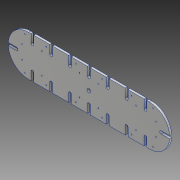
# Autodesk Inventor part: 1313_Former Bottom_V1
Saved by Autodesk Inventor 2020 (Build 240168000, 168)
## iProperties
Created: 2019-09-10
Part Number: 1313_Former Bottom_V1
Material: Aluminum 6061
Document SubType Name: Modeling
Designer: MPI
Density: 2.7 g/cm^3
Appearance: Aluminum - Flat
Mass: 5622.53 g
Surface Area: 6914.04 cm^2
Volume: 5622.53 cm^3
Author: MPI
Autodesk Inventor part; units mm, degrees
ref_plane "Work Plane2" through (0, 0, 0) normal (0, -1, 0) x (1, 0, 0)
sketch "Sketch2" plane through (0, 0, 0) normal (0, -1, 0) x (1, 0, 0)
  line L0 (-432, -146) -> (432, -146)
  line L1 (432, 146) -> (-432, 146)
  line L2 (432, -86) -> (-432, -86) projected
  line L3 (-432, 86) -> (432, 86) projected
  arc A0 (-432, 86) -> (-432, -86) centre (-432, 0) ccw projected
  arc A1 (432, -86) -> (432, 86) centre (432, 0) ccw projected
  arc A2 (432, -146) -> (432, 146) centre (432, 0) ccw
  arc A3 (-432, 146) -> (-432, -146) centre (-432, 0) ccw
  point P0 (0, 0)
  point P1 (480, -91)
  point P2 (480, 91)
  dimension "d11" = 60
  dimension "d12" = 60
  constraints: 4 end point, 4 point on circle, 2 centre point, 2 coincident, 2 tangent, 1 horizontal, 1 parallel, 3 other
extrude "Extrusion2" add sketch "Sketch2" along normal blind 15 contours A3 L1 A2 L0 | L2 A0 L3 A1
ref_plane "Work Plane1" through (0, 7.01, 0) normal (0, 1, 0) x (1, 0, 0)
sketch "Sketch4" plane through (0, 7.01, 0) normal (0, 1, 0) x (1, 0, 0)
  line L0 (-659.0781, -10) -> (-659.0781, 10)
  line L1 (670.9769, 10) -> (670.9769, -10)
  line L2 (-10, 220.6364) -> (10, 220.6364)
  line L3 (-125, -216.3636) -> (-145, -216.3636)
  line L4 (-145, 220.6364) -> (-125, 220.6364)
  line L5 (-260, -216.3636) -> (-280, -216.3636)
  line L6 (-280, 220.6364) -> (-260, 220.6364)
  line L7 (145, -216.3636) -> (125, -216.3636)
  line L8 (125, 220.6364) -> (145, 220.6364)
  line L9 (280, -216.3636) -> (260, -216.3636)
  line L10 (260, 220.6364) -> (280, 220.6364)
  line L11 (395, 220.6364) -> (415, 220.6364)
  line L12 (-432, -86) -> (432, -86) projected
  line L13 (432, 86) -> (-432, 86) projected
  line L14 (395, 86) -> (395, 220.6364)
  line L15 (415, 220.6364) -> (415, 86)
  line L16 (280, -86) -> (280, -216.3636)
  line L17 (260, -216.3636) -> (260, -86)
  line L18 (280, 220.6364) -> (280, 86)
  line L19 (260, 86) -> (260, 220.6364)
  line L20 (145, -86) -> (145, -216.3636)
  line L21 (125, -216.3636) -> (125, -86)
  line L22 (145, 220.6364) -> (145, 86)
  line L23 (125, 86) -> (125, 220.6364)
  line L24 (10, 220.6364) -> (10, 86)
  line L25 (-10, 86) -> (-10, 220.6364)
  line L26 (-125, -86) -> (-125, -216.3636)
  line L27 (-145, -216.3636) -> (-145, -86)
  line L28 (-125, 220.6364) -> (-125, 86)
  line L29 (-145, 86) -> (-145, 220.6364)
  line L30 (-260, -86) -> (-260, -216.3636)
  line L31 (-280, -216.3636) -> (-280, -86)
  line L32 (-260, 220.6364) -> (-260, 86)
  line L33 (-280, 86) -> (-280, 220.6364)
  arc A0 (395, 86) -> (415, 86) centre (405, 86) ccw
  arc A1 (260, 86) -> (280, 86) centre (270, 86) ccw
  arc A2 (125, 86) -> (145, 86) centre (135, 86) ccw
  arc A3 (-10, 86) -> (10, 86) centre (0, 86) ccw
  arc A4 (-145, 86) -> (-125, 86) centre (-135, 86) ccw
  arc A5 (-280, 86) -> (-260, 86) centre (-270, 86) ccw
  arc A6 (-260, -86) -> (-280, -86) centre (-270, -86) ccw
  arc A7 (-125, -86) -> (-145, -86) centre (-135, -86) ccw
  arc A8 (145, -86) -> (125, -86) centre (135, -86) ccw
  arc A9 (280, -86) -> (260, -86) centre (270, -86) ccw
  arc A10 (432, -86) -> (432, 86) centre (432, 0) ccw projected
  arc A11 (518, 10) -> (518, -10) centre (518, 0) ccw
  arc A12 (-518, -10) -> (-518, 10) centre (-518, 0) ccw
  line L34 (-659.0781, 10) -> (-518, 10)
  line L35 (517.4166, 10) -> (670.9769, 10)
  line L36 (670.9769, -10) -> (518, -10)
  line L37 (-518, -10) -> (-659.0781, -10)
  circle A13 centre (-480, 48) radius 3.57
  circle A14 centre (-337.5, 76) radius 3.57
  circle A15 centre (337.5, 76) radius 3.57
  circle A16 centre (480, 48) radius 3.57
  circle A17 centre (480, -48) radius 3.57
  circle A18 centre (337.5, -76) radius 3.57
  circle A19 centre (-337.5, -76) radius 3.57
  circle A20 centre (-480, -48) radius 3.57
  arc A21 (-432, 86) -> (-432, -86) centre (-432, 0) ccw projected
  line L38 (10, -86) -> (10, -216.3636)
  line L39 (-10, -216.3636) -> (-10, -86)
  arc A22 (10, -86) -> (-10, -86) centre (0, -86) ccw
  line L40 (-10, -216.3636) -> (10, -216.3636)
  line L41 (-415, 220.6364) -> (-395, 220.6364)
  line L42 (-395, 220.6364) -> (-395, 86)
  line L43 (-415, 86) -> (-415, 220.6364)
  arc A23 (-415, 86) -> (-395, 86) centre (-405, 86) ccw
  line L44 (415, -216.3636) -> (395, -216.3636)
  line L45 (415, -86) -> (415, -216.3636)
  line L46 (395, -216.3636) -> (395, -86)
  arc A24 (415, -86) -> (395, -86) centre (405, -86) ccw
  line L47 (-395, -216.3636) -> (-415, -216.3636)
  line L48 (-395, -86) -> (-395, -216.3636)
  line L49 (-415, -216.3636) -> (-415, -86)
  arc A25 (-395, -86) -> (-415, -86) centre (-405, -86) ccw
  line L50 (-432, 0) -> (-518, 0)
  circle A26 centre (-67.5, 76) radius 3.57
  circle A27 centre (67.5, 76) radius 3.57
  circle A28 centre (67.5, -76) radius 3.57
  circle A29 centre (-67.5, -76) radius 3.57
  point P0 (480, -91)
  point P1 (480, 91)
  point P2 (-395, 86)
  point P3 (-395, 86)
  dimension "d18" = 20
  dimension "d54" = 76
  dimension "d55" = 48
  dimension "d59" = 48
  dimension "d60" = 76
  dimension "d73" = 7.14
  dimension "d109" = 135
  dimension "d110" = 135
  dimension "d111" = 135
  dimension "d112" = 135
  dimension "d113" = 135
  dimension "d115" = 135
  dimension "d116" = 20
  dimension "d120" = 48
  dimension "d121" = 38
  dimension "d122" = 38
  dimension "d123" = 48
  dimension "d124" = 38
  dimension "d125" = 38
  dimension "d130" = 76
  dimension "d131" = 76
  dimension "d144" = 76
  dimension "d145" = 76
  dimension "d146" = 76
  dimension "d147" = 76
  dimension "d149" = 57.5
  dimension "d150" = 57.5
  dimension "d151" = 57.5
  dimension "d152" = 57.5
  dimension "d153" = 57.5
  dimension "d154" = 57.5
  dimension "d155" = 57.5
  dimension "d156" = 57.5
  constraints: 98 end point, 33 point on circle, 31 parallel, 28 centre point, 25 collinear, 24 tangent, 12 perpendicular, 11 equal radius, 10 horizontal, 3 point on line, 2 vertical, 26 other
  measures "d18" distance of L0.start L0.end
  measures "d54" vertical distance of A15.centre A11.centre
  measures "d55" vertical distance of A11.centre A16.centre
  measures "d59" vertical distance of A17.centre A11.centre
  measures "d60" vertical distance of A18.centre A11.centre
  measures "d73" diameter of A13
  measures "d109" distance between parallel lines of L22 L24
  measures "d110" distance between parallel lines of L18 L22
  measures "d111" distance between parallel lines of L15 L18
  measures "d112" distance between parallel lines of L29 L25
  measures "d113" distance between parallel lines of L33 L29
  measures "d115" distance between parallel lines of L43 L33
  measures "d116" distance of L2.start L2.end
  measures "d120" vertical distance of A20.centre L50.end
  measures "d121" horizontal distance of A20.centre L50.end
  measures "d122" horizontal distance of A13.centre L50.end
  measures "d123" vertical distance of L50.end A13.centre
  measures "d124" horizontal distance of A11.centre A16.centre
  measures "d125" horizontal distance of A11.centre A17.centre
  measures "d130" vertical distance of L50.end A14.centre
  measures "d131" distance from line of L50 A19.centre
  measures "d144" vertical distance of A11.centre A27.centre
  measures "d145" vertical distance of A11.centre A28.centre
  measures "d146" vertical distance of L50.end A26.centre
  measures "d147" vertical distance of L50.end A29.centre
  measures "d149" distance from line of A14.centre L33
  measures "d150" distance from line of L31 A19.centre
  measures "d151" distance from line of A26.centre L28
  measures "d152" distance from line of A29.centre L26
  measures "d153" distance from line of A27.centre L23
  measures "d154" distance from line of A28.centre L21
  measures "d155" distance from line of A15.centre L18
  measures "d156" distance from line of L16 A18.centre
extrude "Extrusion3" cut sketch "Sketch4" against normal through all contours L0 L34 A12 A21 L37 | A21 L50 A12 | A12 L50 A21 | A25 L12 | L12 L48 L47 L49 | L43 L41 L42 L13 | L13 A23 | A6 L12 | L12 L30 L5 L31 | L33 L6 L32 L13 | L13 A5 | A7 L12 | L12 L26 L3 L27 | L29 L4 L28 L13 | L13 A4 | A22 L12 | L12 L38 L40 L39 | L25 L2 L24 L13 | L13 A3 | A8 L12 | L12 L20 L7 L21 | L23 L8 L22 L13 | L13 A2 | A9 L12 | L12 L16 L9 L17 | L19 L10 L18 L13 | L13 A1 | A24 L12 | L12 L45 L44 L46 | L14 L11 L15 L13 | L13 A0 | A11 A10 | A10 A11 L35 L1 L36 | A13 | A14 | A15 | A16 | A17 | A18 | A19 | A20 | A26 | A27 | A28 | A29
ref_plane "Work Plane3" through (0, -15, 0) normal (0, -1, 0) x (1, 0, 0)
sketch "Sketch8" plane through (0, -15, 0) normal (0, -1, 0) x (1, 0, 0)
  circle A0 centre (0, 0) radius 475 construction
  line L0 (-733, 120) -> (746, 120) construction
  line L1 (746, 120) -> (746, -120) construction
  line L2 (746, -120) -> (-733, -120) construction
  line L3 (-733, -120) -> (-733, 120) construction
  circle A1 centre (-459.5922, 120) radius 3.57
  circle A2 centre (-459.5922, -120) radius 3.57
  circle A3 centre (459.5922, 120) radius 3.57
  circle A4 centre (459.5922, -120) radius 3.57
  line L4 (-95, 223) -> (95, 223) construction
  line L5 (95, 223) -> (95, -273) construction
  line L6 (95, -273) -> (-95, -273) construction
  line L7 (-95, -273) -> (-95, 223) construction
  circle A5 centre (-95, 120) radius 3.57
  circle A6 centre (95, 120) radius 3.57
  circle A7 centre (95, -120) radius 3.57
  circle A8 centre (-95, -120) radius 3.57
  circle A9 centre (0, 0) radius 13
  circle A10 centre (0, 0) radius 509.5
  line L8 (-305, 252.8869) -> (-305, -295.4174) construction
  line L9 (305, 244.7236) -> (305, -288.6146) construction
  circle A11 centre (-305, 120) radius 3.57
  circle A12 centre (-305, -120) radius 3.57
  circle A13 centre (305, 120) radius 3.57
  circle A14 centre (305, -120) radius 3.57
  dimension "d78" = 950
  dimension "d79" = 240
  dimension "d80" = 120
  dimension "d81" = 7.14
  dimension "d82" = 7.14
  dimension "d83" = 7.14
  dimension "d84" = 7.14
  dimension "d85" = 190
  dimension "d86" = 95
  dimension "d87" = 7.14
  dimension "d89" = 7.14
  dimension "d91" = 7.14
  dimension "d93" = 7.14
  dimension "d98" = 26
  dimension "d132" = 1019
  dimension "d133" = 210
  dimension "d134" = 210
  dimension "d135" = 7.14
  dimension "d136" = 7.14
  dimension "d137" = 7.14
  dimension "d138" = 7.14
  constraints: 20 end point, 20 point on line, 15 centre point, 4 parallel, 4 point on circle, 3 coincident, 2 horizontal, 2 perpendicular, 2 vertical
  measures "d78" diameter of A0
  measures "d79" distance of L0.end L1.end
  measures "d80" distance from line of point (0, 0) L0
  measures "d81" diameter of A1
  measures "d82" diameter of A2
  measures "d83" diameter of A3
  measures "d84" diameter of A4
  measures "d85" distance of L4.start L4.end
  measures "d86" distance from line of point (0, 0) L7
  measures "d87" diameter of A5
  measures "d89" diameter of A6
  measures "d91" diameter of A7
  measures "d93" diameter of A8
  measures "d98" diameter of A9
  measures "d132" diameter of A10
  measures "d133" distance between parallel lines of L8 L7
  measures "d134" distance between parallel lines of L9 L5
  measures "d135" diameter of A11
  measures "d136" diameter of A12
  measures "d137" diameter of A13
  measures "d138" diameter of A14
extrude "Extrusion5" cut sketch "Sketch8" against normal through all contours A1 | A2 | A3 | A4 | A5 | A6 | A7 | A8 | A9 | A11 | A12 | A13 | A14
body "Solid1"
